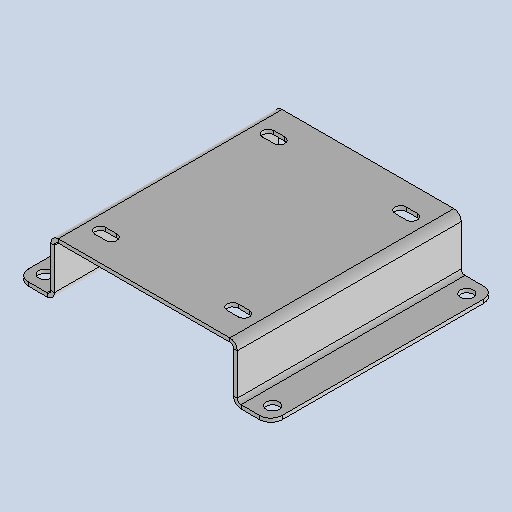
# Autodesk Inventor part: PNS- motor 030 reductor pillar
Saved by Autodesk Inventor 2025.3 (Build 293356030, 356C)
## iProperties
Created: 2025-09-03
Part Number: PNS- motor 030 reductor pillar
Material: Generic
Document SubType Name: Sheet Metal
Designer: admin
Mass: 43.96 g
Surface Area: 455.895 cm^2
Volume: 43.96 cm^3
Density: 1 g/cm^3
Sheet Metal Rule: Default
Sheet Metal Width: 120,000 mm
Sheet Metal Length: 186,096 mm
Sheet Metal Area: 22331,469 mm^2
Appearance: Default
Flat Pattern Width: 12 cm
Flat Pattern Length: 18.6096 cm
Flat Pattern Area: 223.315 cm^2
Author: admin
Autodesk Inventor part; units mm, degrees
ref_plane "YZ Plane" through (0, 0, 0) normal (1, 0, 0) x (0, 1, 0)
ref_plane "XZ Plane" through (0, 0, 0) normal (0, 1, 0) x (-1, 0, 0)
ref_plane "XY Plane" through (0, 0, 0) normal (0, 0, 1) x (1, 0, 0)
sketch "Sketch1" plane through (0, 0, 0) normal (0, 0, 1) x (1, 0, 0)
  line L0 (-50, -60) -> (50, -60)
  line L1 (50, -60) -> (50, 60)
  line L2 (50, 60) -> (-50, 60)
  line L3 (-50, 60) -> (-50, -60)
  line L4 (-50, -60) -> (50, 60) construction
  line L5 (50, -60) -> (-50, 60) construction
  point P0 (0, 0)
  dimension "d0" = 100
  dimension "d1" = 120
  measures "d0" distance of L2.end L1.end
  measures "d1" distance of L1.end L0.end
extrude "Plate1" add sketch "Sketch1" along normal blind 2
sketch "Sketch5" plane through (48, -60, 2) normal (1, 0, 0) x (0, 1, 0)
  line L0 (120, 0) -> (0, 0)
  line L1 (0, 0) -> (0, -30)
  line L2 (0, -30) -> (120, -30)
  line L3 (120, -30) -> (120, 0)
  constraints: 6 end point, 1 horizontal, 1 perpendicular, 1 vertical
edge flange "Flange2" height 30 angle 90 thickness 2 bend radius 2 thickness toward (1, 0, 0) relief tear relief width 2 relief depth 1 corner gap 2 corner form 0 edges at (50, 0, 0) (-50, 0, 0) wall of the first edge with corners at (48, 60, 2) (48, -60, 2) (48, -60, -28) (48, 60, -28)
bend "Bend2"
corner "Corner2"
sketch "Sketch6" plane through (-48, -60, -26) normal (0, 0, -1) x (-1, 0, 0)
  line L0 (0, 120) -> (0, 0)
  line L1 (0, 0) -> (20, 0)
  line L2 (20, 0) -> (20, 120)
  line L3 (20, 120) -> (0, 120)
  constraints: 6 end point, 1 horizontal, 1 perpendicular, 1 vertical
edge flange "Flange3" height 20 angle 90 thickness 2 bend radius 2 thickness toward (0, 0, -1) relief tear relief width 2 relief depth 1 corner gap 2 corner form 0 edges at (-50, 0, -28) (50, 0, -28) wall of the first edge with corners at (-48, 60, -26) (-48, -60, -26) (-68, -60, -26) (-68, 60, -26)
bend "Bend3"
corner "Corner3"
sketch "Sketch7" plane through (0, 0, 2) normal (0, 0, 1) x (1, 0, 0)
  line L0 (-38.5, 45) -> (-32.5, 45) construction
  line L1 (-38.5, 48) -> (-32.5, 48)
  line L2 (-32.5, 42) -> (-38.5, 42)
  arc A0 (-38.5, 48) -> (-38.5, 42) centre (-38.5, 45) ccw
  arc A1 (-32.5, 42) -> (-32.5, 48) centre (-32.5, 45) ccw
  line L3 (0, 0) -> (0, 36.7508)
  line L4 (0, 0) -> (-25.7119, 0)
  line L5 (32.5, 45) -> (38.5, 45) construction
  line L6 (32.5, 48) -> (38.5, 48)
  line L7 (38.5, 42) -> (32.5, 42)
  arc A2 (32.5, 48) -> (32.5, 42) centre (32.5, 45) ccw
  arc A3 (38.5, 42) -> (38.5, 48) centre (38.5, 45) ccw
  line L8 (-38.5, -45) -> (-32.5, -45) construction
  line L9 (-38.5, -42) -> (-32.5, -42)
  line L10 (-32.5, -48) -> (-38.5, -48)
  arc A4 (-38.5, -42) -> (-38.5, -48) centre (-38.5, -45) ccw
  arc A5 (-32.5, -48) -> (-32.5, -42) centre (-32.5, -45) ccw
  line L11 (32.5, -45) -> (38.5, -45) construction
  line L12 (32.5, -42) -> (38.5, -42)
  line L13 (38.5, -48) -> (32.5, -48)
  arc A6 (32.5, -42) -> (32.5, -48) centre (32.5, -45) ccw
  arc A7 (38.5, -48) -> (38.5, -42) centre (38.5, -45) ccw
  point P0 (-35.5, 45)
  point P1 (35.5, 45)
  point P2 (-35.5, -45)
  point P3 (35.5, -45)
  dimension "d42" = 6
  dimension "d43" = 6
  dimension "d50" = 71
  dimension "d51" = 90
  constraints: 36 end point, 16 point on circle, 16 tangent, 8 centre point, 5 horizontal, 4 midpoint, 4 parallel, 3 equal length, 3 equal radius, 2 symmetric about line, 2 vertical alignment, 1 horizontal alignment, 1 vertical
  measures "d42" distance between parallel lines of L2 L1
  measures "d43" distance of L0.start L0.end
  measures "d50" distance of point (35.5, 45) point (-35.5, 45)
  measures "d51" distance of point (-35.5, -45) point (-35.5, 45)
extrude "Cut1" cut sketch "Sketch7" against normal blind 2
sketch "Sketch8" plane through (-68, -60, -26) normal (0, 0, 1) x (1, 0, 0)
  circle A0 centre (7, 112) radius 3.5
  circle A1 centre (7, 8) radius 3.5
  line L0 (16, 120) -> (0, 120) projected
  line L1 (0, 120) -> (0, 0) projected
  line L2 (0, 60) -> (53.6667, 60)
  point P0 (68, 60)
  dimension "d54" = 7
  dimension "d55" = 8
  dimension "d56" = 7
  constraints: 2 centre point, 2 end point, 1 equal radius, 1 horizontal, 1 midpoint, 1 symmetric about line
  measures "d54" diameter of A0
  measures "d55" distance from line of L0 A0.centre
  measures "d56" distance from line of A0.centre L1
extrude "Cut2" cut sketch "Sketch8" against normal blind 2
mirror "Mirror1" about plane through (0, 0, 0) normal (1, 0, 0) of "Cut2"
fillet "Corner Round1" radius 6 4 edges at (-68, -60, -27) (-68, 60, -27) (68, 60, -27) (68, -60, -27)
equation "\"d52\" = Thickness"
equation "\"d57\" = Thickness"
equation "\"d2\" = Thickness"
equation "\"d22\" = BendReliefWidth"
equation "\"d23\" = BendReliefDepth"
equation "\"d24\" = MinimumRemnant"
equation "\"d25\" = TransitionRadius"
equation "\"d28\" = BendRadius"
equation "\"d29\" = CornerReliefSize"
equation "\"d30\" = GapSize"
equation "\"d31\" = JacobiRadiusSize"
equation "\"d32\" = BendReliefWidth"
equation "\"d33\" = BendReliefDepth"
equation "\"d34\" = MinimumRemnant"
equation "\"d35\" = TransitionRadius"
equation "\"d38\" = BendRadius"
equation "\"d39\" = CornerReliefSize"
equation "\"d40\" = GapSize"
equation "\"d41\" = JacobiRadiusSize"
equation "\"BendRadius\" = Thickness"
equation "\"BendReliefWidth\" = Thickness"
equation "\"BendReliefDepth\" = 0.5 * Thickness"
equation "\"CornerReliefSize\" = 4 * Thickness"
equation "\"MinimumRemnant\" = 2 * Thickness"
equation "\"TransitionRadius\" = BendRadius"
equation "\"JacobiRadiusSize\" = BendRadius"
equation "\"GapSize\" = Thickness"
equation "\"Thickness\" = 2"
body "Solid1"
